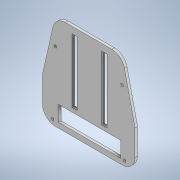
# Autodesk Inventor part: tapa
Saved by Autodesk Inventor 2020 (Build 240168000, 168)
## iProperties
Created: 2020-11-22
Part Number: tapa
Material: Generic
Document SubType Name: Modeling
Designer: michelin
Density: 1 g/cm^3
Appearance: Default
Author: michelin
Autodesk Inventor part; units mm, degrees
ref_plane "YZ Plane" through (0, 0, 0) normal (1, 0, 0) x (0, 1, 0)
ref_plane "XZ Plane" through (0, 0, 0) normal (0, 1, 0) x (-1, 0, 0)
ref_plane "XY Plane" through (0, 0, 0) normal (0, 0, 1) x (1, 0, 0)
sketch "Sketch1" plane through (0, 0, 0) normal (0, 0, 1) x (1, 0, 0)
  line L0 (-90.4669, 29.5677) -> (-90.4669, 104.3985)
  circle A0 centre (-65.3126, 164.3997) radius 2.5
  circle A1 centre (64.5331, 164.2566) radius 2.5
  circle A2 centre (69.5331, 39.5677) radius 2.5
  circle A3 centre (-70.4669, 39.5677) radius 2.5
  line L1 (-59.3477, 39.5677) -> (62.0331, 39.5677)
  line L2 (62.0331, 39.5677) -> (62.0331, 69.7525)
  line L3 (62.0331, 69.7525) -> (-59.3477, 69.7525)
  line L4 (-59.3477, 69.7525) -> (-59.3477, 39.5677)
  line L5 (25.2356, 77.4734) -> (35.0999, 77.4734)
  line L6 (35.0999, 77.4734) -> (35.0999, 201.5575)
  line L7 (35.0999, 201.5575) -> (25.2356, 201.5575)
  line L8 (25.2356, 201.5575) -> (25.2356, 77.4734)
  line L9 (-32.8575, 77.7729) -> (-22.9932, 77.7729)
  line L10 (-22.9932, 77.7729) -> (-22.9932, 201.8569)
  line L11 (-22.9932, 201.8569) -> (-32.8575, 201.8569)
  line L12 (-32.8575, 201.8569) -> (-32.8575, 77.7729)
  line L13 (-90.4669, 29.5677) -> (89.4944, 29.5677)
  line L14 (-65.4669, 214.4401) -> (64.5331, 214.4401)
  line L15 (-90.4669, 104.3985) -> (-65.4669, 214.4401)
  line L16 (64.5331, 214.4401) -> (89.4944, 104.2566)
  line L17 (89.4944, 104.2566) -> (89.4944, 29.5677)
  constraints: 36 end point, 6 parallel, 5 horizontal, 4 centre point, 3 perpendicular, 1 vertical
extrude "Extrusion1" add sketch "Sketch1" along normal blind 5
fillet "Fillet1" radius 25 4 edges at (64.5331, 214.4401, 2.5) (-65.4669, 214.4401, 2.5) (-90.4669, 29.5677, 2.5) (89.4944, 29.5677, 2.5)
body "Solid1"
